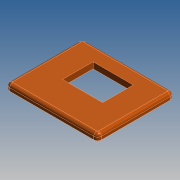
# Autodesk Inventor part: A2_TopCase
Saved by Autodesk Inventor 2020.2 (Build 242310000, 310)
## iProperties
Created: 2021-08-29
Part Number: A2_TopCase
Material: Plastique ABS
Document SubType Name: Modeling
Designer: Samy Francelet
Density: 1.06 g/cm^3
Appearance: Lisse - Orange clair
Author: Samy Francelet
Autodesk Inventor part; units mm, degrees
ref_plane "YZ Plane" through (0, 0, 0) normal (1, 0, 0) x (0, 1, 0)
ref_plane "XZ Plane" through (0, 0, 0) normal (0, 1, 0) x (-1, 0, 0)
ref_plane "XY Plane" through (0, 0, 0) normal (0, 0, 1) x (1, 0, 0)
sketch "Esquisse2" plane through (0, 0, 0) normal (0, 0, 1) x (1, 0, 0)
  line L0 (-85.4497, 0) -> (85.4497, 0) construction
  line L1 (0, -71.4497) -> (0, 71.4497) construction
  line L2 (-55, -50) -> (55, -50)
  line L3 (60, -45) -> (60, 45)
  line L4 (55, 50) -> (-55, 50)
  line L5 (-60, 45) -> (-60, -45)
  line L6 (-60, -50) -> (60, 50) construction
  line L7 (60, -50) -> (-60, 50) construction
  arc A0 (-55, 50) -> (-60, 45) centre (-55, 45) ccw
  arc A1 (-60, -45) -> (-55, -50) centre (-55, -45) ccw
  arc A2 (55, -50) -> (60, -45) centre (55, -45) ccw
  arc A3 (60, 45) -> (55, 50) centre (55, 45) ccw
  point P0 (0, 0)
  dimension "d0" = 120
  dimension "d1" = 100
  dimension "d2" = 5
  constraints: 12 end point, 8 point on circle, 8 point on line, 8 tangent, 4 centre point, 3 equal radius, 2 midpoint, 2 parallel, 1 horizontal, 1 perpendicular
  measures "d0" distance of L7.end L6.end
  measures "d1" distance of L6.end L7.start
  measures "d2" radius of A0
extrude "Extrusion1" add sketch "Esquisse2" along normal blind 8
fillet "Congé1" radius 4 8 edges at (58.5355, -48.5355, 8) (60, 0, 8) (58.5355, 48.5355, 8) (0, 50, 8) (-58.5355, 48.5355, 8) (-60, 0, 8) (-58.5355, -48.5355, 8) (0, -50, 8)
sketch "Esquisse3" plane through (0, 0, 8) normal (0, 0, 1) x (1, 0, 0)
  line L0 (-84, 0) -> (84, 0) construction
  line L1 (0, -70) -> (0, 70) construction
  line L2 (55, 50) -> (-55, 50) construction
  line L3 (-60, 45) -> (-60, -45) construction
  line L4 (-60, 50) -> (-26, 50) construction
  line L5 (-26, 50) -> (-26, 30) construction
  line L6 (-26, 30) -> (-60, 30) construction
  line L7 (-60, 30) -> (-60, 50) construction
  line L8 (-26, 30) -> (26.5, 30)
  line L9 (26.5, 30) -> (26.5, -10)
  line L10 (26.5, -10) -> (-26, -10)
  line L11 (-26, -10) -> (-26, 30)
  point P0 (0, 0)
  dimension "d6" = 34
  dimension "d7" = 20
  dimension "d8" = 52.5
  dimension "d9" = 40
  constraints: 16 end point, 4 parallel, 2 collinear, 2 horizontal, 2 perpendicular
  measures "d6" distance of L5.end L6.end
  measures "d7" distance of L4.end L5.end
  measures "d8" distance of L9.end L10.end
  measures "d9" distance of L8.end L9.end
extrude "Extrusion2" cut sketch "Esquisse3" against normal through all
